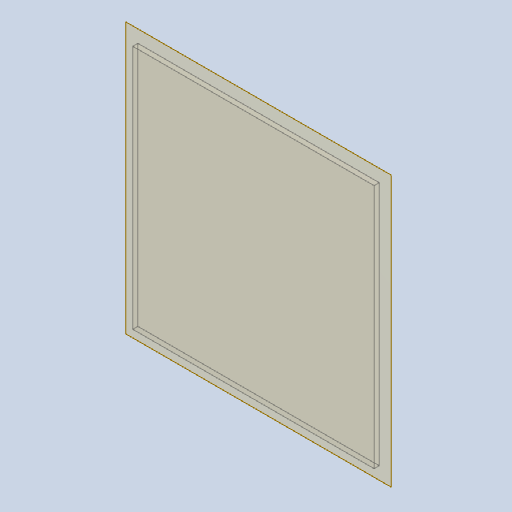
# Autodesk Inventor part: Lid
Saved by Autodesk Inventor 2022.2 (Build 262287000, 287)
## iProperties
Created: 2022-01-15
Part Number: Lid
Material: Polycarbonate, Clear
Document SubType Name: Modeling
Designer: siwat
Density: 1.2 g/cm^3
Appearance: Polycarbonate - Clear
Author: siwat
Autodesk Inventor part; units mm, degrees
ref_plane "YZ Plane" through (0, 0, 0) normal (1, 0, 0) x (0, 1, 0)
ref_plane "XZ Plane" through (0, 0, 0) normal (0, 1, 0) x (-1, 0, 0)
ref_plane "XY Plane" through (0, 0, 0) normal (0, 0, 1) x (1, 0, 0)
ref_plane "Work Plane1" through (0, 0, 0) normal (0, 0, 1) x (1, 0, 0)
sketch "Sketch1" plane through (0, 0, 0) normal (0, 0, 1) x (1, 0, 0)
  line L0 (71.2978, -72.4006) -> (-71.2977, -72.4006)
  line L1 (-71.2977, -72.4006) -> (-71.2977, 72.4006)
  line L2 (-71.2977, 72.4006) -> (71.2978, 72.4006)
  line L3 (71.2978, 72.4006) -> (71.2978, -72.4006)
  point P0 (0, 0)
  constraints: 8 end point, 2 parallel, 1 horizontal, 1 perpendicular
extrude "Extrusion1" add sketch "Sketch1" along normal blind 3
body "Solid1"
